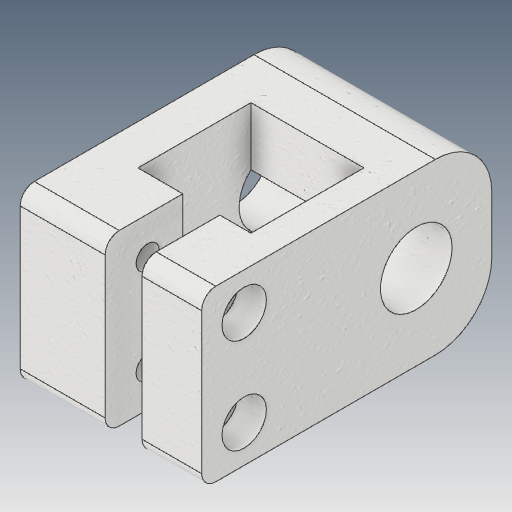
# Autodesk Inventor part: 3d printed motor shaft block for base v1
Saved by Autodesk Inventor 2018 (Build 220112000, 112)
## iProperties
Created: 2019-10-10
Part Number: 3d printed motor shaft block for base v1
Material: Generic
Document SubType Name: Modeling
Designer: Matt
Density: 1 g/cm^3
Appearance: custom powder coated white1
Author: Matt
Autodesk Inventor part; units mm, degrees
ref_plane "YZ Plane" through (0, 0, 0) normal (1, 0, 0) x (0, 1, 0)
ref_plane "XZ Plane" through (0, 0, 0) normal (0, 1, 0) x (-1, 0, 0)
ref_plane "XY Plane" through (0, 0, 0) normal (0, 0, 1) x (1, 0, 0)
sketch "Sketch1" plane through (0, 0, 0) normal (0, 1, 0) x (-1, 0, 0)
  arc A0 (5.6966, -10.4681) -> (3.0156, -10.4681) centre (4.3561, -12.7) ccw projected
  line L0 (17.0561, -25.4) -> (-8.3439, -25.4)
  line L1 (-8.3439, -25.4) -> (-8.3439, 0)
  line L2 (17.0561, 0) -> (17.0561, -25.4)
  line L3 (17.0561, -25.4) -> (-8.3439, 0) construction
  line L4 (-8.3439, -25.4) -> (17.0561, 0) construction
  line L5 (-14.7304, 17.477) -> (-14.7304, -47.796)
  line L6 (-14.7304, -47.796) -> (26.0883, -47.796)
  line L7 (26.0883, -47.796) -> (26.0883, 17.477)
  line L8 (-1.3293, 0) -> (-1.3293, 17.477)
  line L9 (6.9778, 17.477) -> (6.9778, 0)
  line L10 (-8.3439, 0) -> (-1.3293, 0)
  line L11 (6.9778, 0) -> (17.0561, 0)
  line L12 (26.0883, 17.477) -> (6.9778, 17.477)
  line L13 (-1.3293, 17.477) -> (-14.7304, 17.477)
  point P0 (0, 0)
  dimension "d0" = 25.4
  dimension "d1" = 25.4
  constraints: 28 end point, 7 parallel, 3 horizontal, 3 perpendicular, 2 midpoint, 1 collinear
  measures "d0" distance of L1.end L2.start
  measures "d1" distance of L0.end L1.end
extrude "Extrusion1" add sketch "Sketch1" along normal mid plane 38.1
sketch "Sketch2" plane through (14.7304, -19.05, -47.796) normal (1, 0, 0) x (0, 0, -1)
  arc A0 (-22.6007, 24.7617) -> (-22.396, 13.1445) centre (-16.9992, 19.05) ccw projected
  circle A1 centre (-16.9992, 19.05) radius 8
  circle A2 centre (-16.9992, 19.05) radius 8.0635
  point P0 (-47.796, 19.05)
  dimension "d4" = 0.0635
  constraints: 2 centre point, 1 coincident
  measures "d4" radial gap between concentric circles of A1 A2
extrude "Extrusion2" cut sketch "Sketch2" against normal through all contours A1 A0 | A2
fillet "Fillet1" radius 12.7 2 edges at (-5.6789, -19.05, -47.796) (-5.6789, 19.05, -47.796)
fillet "Fillet2" radius 3.175 4 edges at (8.0299, 19.05, 17.477) (-16.533, 19.05, 17.477) (-16.533, -19.05, 17.477) (8.0299, -19.05, 17.477)
sketch "Sketch3" plane through (14.7304, -6.35, -47.796) normal (1, 0, 0) x (0, 0, -1)
  circle A0 centre (-16.9992, 6.35) radius 8.0635 projected
  arc A1 (-65.2731, -9.525) -> (-62.0981, -12.7) centre (-62.0981, -9.525) ccw projected
  line L0 (-12.7, -12.7) -> (-62.0981, -12.7) projected
  arc A2 (-12.7, -12.7) -> (0, 0) centre (-12.7, 0) ccw projected
  line L1 (0, 0) -> (0, 12.7) projected
  arc A3 (0, 12.7) -> (-12.7, 25.4) centre (-12.7, 12.7) ccw projected
  line L2 (-62.0981, 25.4) -> (-12.7, 25.4) projected
  arc A4 (-62.0981, 25.4) -> (-65.2731, 22.225) centre (-62.0981, 22.225) ccw projected
  line L3 (-65.2731, -9.525) -> (-65.2731, 22.225) projected
  line L4 (-48.1725, 17.0318) -> (-55.7015, 17.0318) construction
  line L5 (-55.7015, 17.0318) -> (-55.7015, -4.3318) construction
  line L6 (-55.7015, -4.3318) -> (-48.1725, -4.3318) construction
  line L7 (-48.1725, -4.3318) -> (-48.1725, 17.0318) construction
  line L8 (-48.1725, 17.0318) -> (-55.7015, -4.3318) construction
  line L9 (-55.7015, 17.0318) -> (-48.1725, -4.3318) construction
  circle A5 centre (-55.7015, 17.0318) radius 2.625
  circle A6 centre (-55.7015, -4.3318) radius 2.625
  point P0 (-47.796, 6.35)
  point P1 (-51.937, 6.35)
  dimension "d9" = 5.25
  dimension "d10" = 5.25
  constraints: 12 end point, 2 centre point, 2 coincident, 2 midpoint, 2 parallel, 1 horizontal, 1 perpendicular
  measures "d9" diameter of A5
  measures "d10" diameter of A6
extrude "Extrusion3" cut sketch "Sketch3" against normal through all contours A5 | A6
sketch "Sketch4" plane through (-26.0883, -6.35, -47.796) normal (-1, 0, 0) x (0, 0, 1)
  circle A0 centre (55.7015, 17.0318) radius 2.625 projected
  circle A1 centre (55.7015, -4.3318) radius 2.625 projected
  circle A2 centre (16.9992, 6.35) radius 8.0635 projected
  arc A3 (62.0981, -12.7) -> (65.2731, -9.525) centre (62.0981, -9.525) ccw projected
  line L0 (65.2731, -9.525) -> (65.2731, 22.225) projected
  arc A4 (65.2731, 22.225) -> (62.0981, 25.4) centre (62.0981, 22.225) ccw projected
  line L1 (12.7, 25.4) -> (62.0981, 25.4) projected
  arc A5 (12.7, 25.4) -> (0, 12.7) centre (12.7, 12.7) ccw projected
  line L2 (0, 0) -> (0, 12.7) projected
  arc A6 (0, 0) -> (12.7, -12.7) centre (12.7, 0) ccw projected
  line L3 (62.0981, -12.7) -> (12.7, -12.7) projected
  line L4 (60.3203, 17.0318) -> (58.0109, 13.0318)
  line L5 (58.0109, 13.0318) -> (53.3921, 13.0318)
  line L6 (53.3921, 13.0318) -> (51.0827, 17.0318)
  line L7 (51.0827, 17.0318) -> (53.3921, 21.0318)
  line L8 (53.3921, 21.0318) -> (58.0109, 21.0318)
  line L9 (58.0109, 21.0318) -> (60.3203, 17.0318)
  line L10 (60.3203, -4.3318) -> (58.0109, -8.3318)
  line L11 (58.0109, -8.3318) -> (53.3921, -8.3318)
  line L12 (53.3921, -8.3318) -> (51.0827, -4.3318)
  line L13 (51.0827, -4.3318) -> (53.3921, -0.3318)
  line L14 (53.3921, -0.3318) -> (58.0109, -0.3318)
  line L15 (58.0109, -0.3318) -> (60.3203, -4.3318)
  point P0 (47.796, 6.35)
  dimension "d13" = 8
  dimension "d14" = 8
  constraints: 24 end point, 2 coincident, 26 other
  measures "d13" distance between parallel lines of L13 L10
  measures "d14" distance between parallel lines of L7 L4
extrude "Extrusion4" cut sketch "Sketch4" against normal blind 12.7 contours L4 L5 L6 L7 L8 L9 | L10 L11 L12 L13 L14 L15
sketch "Sketch5" plane through (14.7304, -6.35, -47.796) normal (1, 0, 0) x (0, 0, -1)
  circle A0 centre (-55.7015, 17.0318) radius 2.625 projected
  circle A1 centre (-55.7015, -4.3318) radius 2.625 projected
  circle A2 centre (-16.9992, 6.35) radius 8.0635 projected
  arc A3 (-65.2731, -9.525) -> (-62.0981, -12.7) centre (-62.0981, -9.525) ccw projected
  line L0 (-12.7, -12.7) -> (-62.0981, -12.7) projected
  arc A4 (-12.7, -12.7) -> (0, 0) centre (-12.7, 0) ccw projected
  line L1 (0, 0) -> (0, 12.7) projected
  arc A5 (0, 12.7) -> (-12.7, 25.4) centre (-12.7, 12.7) ccw projected
  line L2 (-62.0981, 25.4) -> (-12.7, 25.4) projected
  arc A6 (-62.0981, 25.4) -> (-65.2731, 22.225) centre (-62.0981, 22.225) ccw projected
  line L3 (-65.2731, -9.525) -> (-65.2731, 22.225) projected
  circle A7 centre (-55.7015, -4.3318) radius 2.625 projected
  circle A8 centre (-55.7015, -4.3318) radius 5
  circle A9 centre (-55.7015, 17.0318) radius 5
  point P0 (-47.796, 6.35)
  dimension "d17" = 10
  dimension "d18" = 10
  constraints: 2 centre point, 2 coincident
  measures "d17" diameter of A8
  measures "d18" diameter of A9
extrude "Extrusion5" cut sketch "Sketch5" against normal blind 6.35 contours A8 | A9
body "Solid1"
